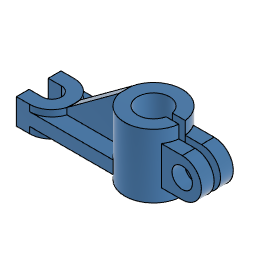
Exercise-7 v1 (Autodesk Fusion 360 design; units mm, degrees)
Autodesk Fusion 360 part; units mm, degrees
sketch "Sketch1" plane through (0, 0, 0) normal (0, 0, 1) x (1, 0, 0)
  line L0 (30.8579, -17.5) -> (-45, -17.5)
  line L1 (-45, 17.5) -> (30.8579, 17.5)
  line L2 (-34.6227, 7.5) -> (-45, 7.5)
  line L3 (-45, -7.5) -> (-34.6227, -7.5)
  line L4 (67.3607, -2.5) -> (57.2474, -2.5)
  line L5 (57.2474, 2.5) -> (67.3607, 2.5)
  line L6 (23.0626, 5) -> (-17.8522, 5)
  line L7 (-17.8522, -5) -> (23.0626, -5)
  arc A0 (-34.6227, -17.5) -> (-34.6227, 17.5) centre (-34.6227, 0) ccw
  line L8 (-45, -17.5) -> (-45, -7.5)
  line L9 (-45, 7.5) -> (-45, 17.5)
  arc A1 (-34.6227, -7.5) -> (-34.6227, 7.5) centre (-34.6227, 0) ccw
  arc A2 (67.3607, 2.5) -> (67.3607, -2.5) centre (45, 0) ccw
  arc A3 (57.2474, 2.5) -> (57.2474, -2.5) centre (45, 0) ccw
  dimension "d2" = 35
  dimension "d3" = 15
  dimension "d4" = 35
  dimension "d5" = 25
  dimension "d6" = 45
  dimension "d8" = 15
  constraint horizontal L0
  constraint perpendicular L0 L8
  constraint parallel L0 L1
  constraint concentric A0 A1
  constraint concentric A2 A3
  constraint horizontal L2
  constraint horizontal L3
  constraint horizontal L4
  constraint parallel L4 L5
  constraint horizontal L6
  constraint parallel L6 L7
  constraint collinear L8 L9
  constraint coincident L1 A0.end
  constraint coincident L0 A0.start
  constraint coincident A0 L6.end
  constraint coincident A0 L7.start
  constraint coincident L6.start A2
  constraint coincident L7.end A2
  constraint coincident L1.end A2
  constraint coincident L0.start A2
  measures "d2" distance of L0.end L1.start
  measures "d3" diameter of A1
  measures "d4" diameter of A0
  measures "d5" diameter of A3
  measures "d6" diameter of A2
  measures "d8" distance of L2.start L3.end
extrude "Extrude1" add sketch "Sketch1" along normal mid plane 10 contours L0 L7 A0 A2 | L6 L7 A0 A2 | L1 L6 A0 A2 makes body 1
extrude "Extrude2" add sketch "Sketch1" along normal mid plane 20 contours L0 L1 L2 L3 A0 L8 L9 A1 bodies 1
extrude "Extrude3" add sketch "Sketch1" along normal blind 40 and the other way blind 10 contours L4 L5 A2 A3 bodies 1
extrude "Extrude4" add sketch "Sketch1" along normal blind 40 contours L6 L7 A0 A2 bodies 1
sketch "Sketch2" plane through (0, -5, 0) normal (0, -1, 0) x (1, 0, 0)
  line L0 (-17.8522, 5) -> (23.0626, 5)
  line L1 (23.0626, 5) -> (23.0626, 40)
  line L2 (23.0626, 40) -> (-17.8522, 40)
  line L3 (-17.8522, 40) -> (-17.8522, 10)
  line L4 (-17.8522, 10) -> (-17.8522, 5)
  line L5 (-17.8522, 10) -> (23.0626, 40)
  line L6 (23.0626, 40) -> (-17.8522, 40)
  line L7 (-17.8522, 40) -> (-17.8522, 10)
  constraint coincident L3.end L4.start
  constraint coincident L1.end L2.start
  constraint coincident L2.end L3.start
extrude "Extrude5" cut sketch "Sketch2" against normal blind 40 contours L2 L3 L5 L6 L7 bodies 1
sketch "Sketch3" plane through (0, 0, 0) normal (0, 1, 0) x (1, 0, 0)
  circle A0 centre (80, -15) radius 8
  line L0 (80, -30) -> (50, -30)
  line L1 (50, -30) -> (50, 0)
  line L2 (50, 0) -> (80, 0)
  line L3 (80, 0) -> (80, -30)
  arc A1 (80, -30) -> (80, 0) centre (80, -15) ccw
  point P0 (-45, 10)
  point P1 (67.3607, 10)
  dimension "d25" = 16
  dimension "d26" = 30
  dimension "d27" = 30
  dimension "d28" = 125
  dimension "d29" = 25
  constraint concentric A0 A1
  constraint horizontal L0
  constraint vertical L1
  constraint horizontal L2
  constraint vertical L3
  measures "d25" diameter of A0
  measures "d26" diameter of A1
  measures "d27" distance of L0.start L2.end
  measures "d28" distance of L3 P0
  measures "d29" vertical distance of A0.centre P1
extrude "Extrude6" add sketch "Sketch3" along normal blind 10 from surface at 2.5 separate body contours A0 L3 A1 | A0 L0 L1 L2 L3 makes body 2
combine "Combine1" operation cut target body 2 tool bodies 1 keep tools makes body 3 at (57.1207, 3.0559, 10)
delete_body "RemoveBody1" bodies 3
mirror "Mirror1" about plane through (0, 0, 0) normal (0, 1, 0) of "Extrude6" makes body 4
combine "Combine2" operation cut target body 4 tool bodies 1 keep tools makes body 5 at (57.1207, -3.0559, 20)
delete_body "RemoveBody2" bodies 5
combine "Combine3" operation add target body 1 tool bodies 2 4 keep tools
